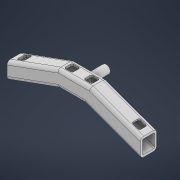
# Autodesk Inventor part: Fahrwerk_bogie
Saved by Autodesk Inventor 2021 (Build 250183000, 183)
## iProperties
Created: 2020-12-29
Part Number: Fahrwerk_bogie
Material: Generisch
Document SubType Name: Modeling
Designer: laure
Density: 1 g/cm^3
Appearance: Vorgabe
Author: laure
Autodesk Inventor part; units mm, degrees
ref_plane "YZ Plane" through (0, 0, 0) normal (1, 0, 0) x (0, 1, 0)
ref_plane "XZ Plane" through (0, 0, 0) normal (0, 1, 0) x (-1, 0, 0)
ref_plane "XY Plane" through (0, 0, 0) normal (0, 0, 1) x (1, 0, 0)
sketch "Skizze1" plane through (0, 0, 0) normal (0, 0, 1) x (1, 0, 0)
  line L0 (-20, 10) -> (20, 10)
  line L1 (-20, 10) -> (-82.019713, -12.573329)
  line L2 (-20, 10) -> (46, 10) construction
  line L3 (-70.548184, -28.95637) -> (-18.465985, -10)
  line L4 (20, 10) -> (82.019713, -12.573329)
  line L5 (20, 10) -> (86, 10) construction
  line L6 (82.019713, -34.868517) -> (13.694024, -10)
  line L7 (-18.465985, -10) -> (13.694024, -10)
  line L8 (-82.019713, -12.573329) -> (-82.019713, -33.131665)
  line L9 (-82.019713, -33.131665) -> (-70.548184, -28.95637)
  line L10 (82.019713, -12.573329) -> (82.019713, -34.868517)
  line L11 (0, 18.973703) -> (0, -43.84222)
  line L12 (-115.623656, 0) -> (119.603943, 0)
  point P0 (0, 0)
  dimension "d0" = 40
  dimension "d3" = 66
  dimension "d5" = 20
  dimension "d7" = 66
  dimension "d8" = 20
  dimension "d84" = 20
  dimension "d85" = 20
  dimension "d87" = 10
  dimension "d89" = 20
  constraints: 22 end point, 4 horizontal, 2 equal length, 2 vertical, 1 point on line, 2 other
  measures "d0" distance of L0.start L0.end
  measures "d3" distance of L0.start L1.end
  measures "d5" distance of L1.end L3.start
  measures "d7" distance of L0.end L4.end
  measures "d8" angle of L4 L5
  measures "d84" angle of L12 L3
  measures "d85" angle of L12 L6
  measures "d87" distance between parallel lines of L0 L12
  measures "d89" angle of L1 L0
extrude "Extrusion1" add sketch "Skizze1" along normal blind 20
sketch "Skizze2" plane through (0, 0, 0) normal (0, 0, -1) x (-1, 0, 0)
  circle A0 centre (0, 0) radius 4.875
  dimension "d11" = 9.75
  constraints: 1 centre point, 1 coincident
  measures "d11" diameter of A0
fillet "Rundung3" radius 4 14 edges at (-51.0099, -1.2867, 20) (-51.0099, -1.2867, 0) (-44.5071, -19.4782, 20) (-76.2839, -31.044, 20) (-44.5071, -19.4782, 0) (-76.2839, -31.044, 0) (-2.386, -10, 0) (-2.386, -10, 20) (0, 10, 0) (51.0099, -1.2867, 0) (47.8569, -22.4343, 0) (47.8569, -22.4343, 20) (0, 10, 20) (51.0099, -1.2867, 20)
shell "Wandung3" thickness 2.6 removed faces 2 at (-82.019713, -24.859983, 13.333333) at (82.019713, -21.423962, 13.333333)
extrude "Extrusion7" add sketch "Skizze2" along normal mid plane 40
sketch "Skizze6" plane through (-82.019713, -12.573329, 16) normal (-0.3420201, 0.9396926, 0) x (0.9396926, 0.3420201, 0)
  line L0 (7, 11) -> (17, 11)
  line L1 (17, 11) -> (17, 1)
  line L2 (17, 1) -> (7, 1)
  line L3 (7, 1) -> (7, 11)
  line L4 (0, 12) -> (0, 0) projected
  line L5 (0, 12) -> (66, 12) projected
  point P0 (81.373651, 16)
  dimension "d51" = 10
  dimension "d52" = 10
  dimension "d53" = 7
  dimension "d54" = 1
  constraints: 8 end point, 2 parallel, 1 horizontal, 1 perpendicular
  measures "d51" distance of L1.end L2.end
  measures "d52" distance of L0.end L1.end
  measures "d53" distance between parallel lines of L3 L4
  measures "d54" distance between parallel lines of L5 L0
extrude "Extrusion8" cut sketch "Skizze6" against normal blind 3
sketch "Skizze7" plane through (20, 10, 16) normal (0.3420201, 0.9396926, 0) x (0.9396926, -0.3420201, 0)
  line L0 (59, 1) -> (49, 1)
  line L1 (49, 1) -> (49, 11)
  line L2 (49, 11) -> (59, 11)
  line L3 (59, 11) -> (59, 1)
  line L4 (66, 12) -> (66, 0) projected
  line L5 (66, 0) -> (0, 0) projected
  point P0 (-15.373651, 16)
  dimension "d57" = 10
  dimension "d58" = 10
  dimension "d59" = 7
  dimension "d60" = 1
  constraints: 8 end point, 2 parallel, 1 horizontal, 1 perpendicular
  measures "d57" distance of L1.end L2.end
  measures "d58" distance of L0.end L1.end
  measures "d59" distance between parallel lines of L4 L3
  measures "d60" distance between parallel lines of L5 L0
extrude "Extrusion9" cut sketch "Skizze7" against normal blind 3
sketch "Skizze8" plane through (-20, 10, 4) normal (0, 1, 0) x (1, 0, 0)
  line L0 (3, -1) -> (13, -1)
  line L1 (13, -1) -> (13, -11)
  line L2 (13, -11) -> (3, -11)
  line L3 (3, -11) -> (3, -1)
  line L4 (0, 0) -> (40, 0) projected
  line L5 (0, 0) -> (0, -12) projected
  line L6 (27, -1) -> (37, -1)
  line L7 (37, -1) -> (37, -11)
  line L8 (37, -11) -> (27, -11)
  line L9 (27, -11) -> (27, -1)
  line L10 (40, 0) -> (40, -12) projected
  point P0 (20, 4)
  dimension "d63" = 10
  dimension "d64" = 10
  dimension "d65" = 1
  dimension "d66" = 3
  dimension "d67" = 10
  dimension "d68" = 10
  dimension "d69" = 1
  dimension "d70" = 3
  constraints: 16 end point, 4 parallel, 2 horizontal, 2 perpendicular
  measures "d63" distance of L1.end L2.end
  measures "d64" distance of L0.end L1.end
  measures "d65" distance between parallel lines of L4 L0
  measures "d66" distance between parallel lines of L5 L3
  measures "d67" distance of L7.end L8.end
  measures "d68" distance of L6.end L7.end
  measures "d69" distance between parallel lines of L4 L6
  measures "d70" distance between parallel lines of L10 L7
extrude "Extrusion10" cut sketch "Skizze8" against normal blind 3
fillet "Rundung7" radius 2 16 edges at (-65.6003, -7.9806, 15) (-74.9972, -11.4008, 15) (-74.9972, -11.4008, 5) (-65.6003, -7.9806, 5) (17, 8.7, 5) (-7, 8.7, 5) (7, 8.7, 15) (-17, 8.7, 15) (-17, 8.7, 5) (17, 8.7, 15) (-7, 8.7, 15) (7, 8.7, 5) (65.6003, -7.9806, 5) (74.9972, -11.4008, 15) (74.9972, -11.4008, 5) (65.6003, -7.9806, 15)
